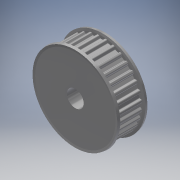
# Autodesk Inventor part: Poulie_stepper
Saved by Autodesk Inventor 2017 (Build 210142000, 142)
## iProperties
Created: 2018-02-01
Part Number: Poulie_stepper
Material: Steel
Document SubType Name: Modeling
Designer: sasha
Density: 1 g/cm^3
Appearance: Steel
CustomPartVersion: 1
Author: sasha
Autodesk Inventor part; units mm, degrees
ref_plane "YZ Plane" through (0, 0, 0) normal (1, 0, 0) x (0, 1, 0)
ref_plane "XZ Plane" through (0, 0, 0) normal (0, 1, 0) x (-1, 0, 0)
ref_plane "XY Plane" through (0, 0, 0) normal (0, 0, 1) x (1, 0, 0)
sketch "Esquisse de poulie" plane through (0, 0, 0) normal (0, 0, 1) x (1, 0, 0)
  circle A0 centre (0, 0) radius 12.7324 construction
  circle A1 centre (0, 0) radius 12.4324
  circle A2 centre (0, 0) radius 11.6824
  line L0 (-0.8608, 12.4026) -> (-0.525, 11.6824)
  line L1 (-0.525, 11.6824) -> (0.525, 11.6824)
  line L2 (0.525, 11.6824) -> (0.8608, 12.4026)
  line L3 (0, 0) -> (0, 12.4324) construction
  point P0 (0, 11.6824)
  dimension "d0" = 25.4648
  dimension "d1" = 0.3
  dimension "d2" = 0.75
  dimension "d3" = 50
  dimension "d4" = 1.05
  constraints: 8 end point, 3 coincident, 3 point on circle, 2 centre point, 1 horizontal, 1 midpoint, 1 point on line, 1 vertical, 1 vertical alignment, 3 other
  measures "d0" diameter of A0
  measures "d1" radial gap between concentric circles of A0 A1
  measures "d3" angle of L2 L0
  measures "d4" distance of L0.end L1.end
extrude "Corps de base" add sketch "Esquisse de poulie" along normal mid plane 7.5 contours A2 | A1 L0 L1 L2 | L2 L1 L0 A1
extrude "Dent" cut sketch "Esquisse de poulie" along normal through all both and the other way through all contours L2 L1 L0 A1 picked at (0, 12.1802)
fillet "Fillet" radius 0.2 2 edges at (0.525, 11.6824, 0) (-0.525, 11.6824, 0)
fillet "Fillet" radius 0.3 4 edges at (-0.8608, 12.4026, 1.875) (-0.8608, 12.4026, -1.875) (0.8608, 12.4026, 1.875) (0.8608, 12.4026, -1.875)
pattern_circular "Dents" count 32 over 360 about axis through (0, 0, -10) along (0, 0, 1) of "Dent", "Fillet"
pulley flange "Bride gauche" diameter 24.8648 height 0.8 thickness 0.8 bend angle 10 centre (0, 0, -3.75) toward (0, 0, -1)
pulley flange "Bride droite" diameter 24.8648 height 0.8 thickness 0.8 bend angle 10 centre (0, 0, 3.75) toward (0, 0, 1)
sketch "Esquisse2" plane through (0, 0, 4.55) normal (0, 0, 1) x (1, 0, 0)
  point P0 (0, 0)
  point P1 (0, 0)
  constraints: 1 coincident
hole "Perçage1" at (0, 0, 4.55) direction (0, 0, -1) diameter 5.2 end through all
equation "\"d1\" = da_a"
equation "\"d2\" = da_hg"
equation "\"d3\" = 2 * da_fi"
equation "\"d4\" = da_bw"
equation "\"d5\" = da_bf"
equation "\"d7\" = da_bf"
equation "\"d9\" = da_rb"
equation "\"d10\" = da_rt"
equation "\"da_pb\" = 2.5"
equation "\"da_fi\" = 25deg"
equation "\"da_hg\" = 0.75"
equation "\"da_bw\" = 1.05"
equation "\"da_rb\" = 0.2"
equation "\"da_rt\" = 0.3"
equation "\"da_a\" = 0.3"
equation "\"da_bf\" = 7.5"
equation "\"da_wf\" = 0.8"
equation "\"da_hf\" = 0.8"
body "Solid1"
